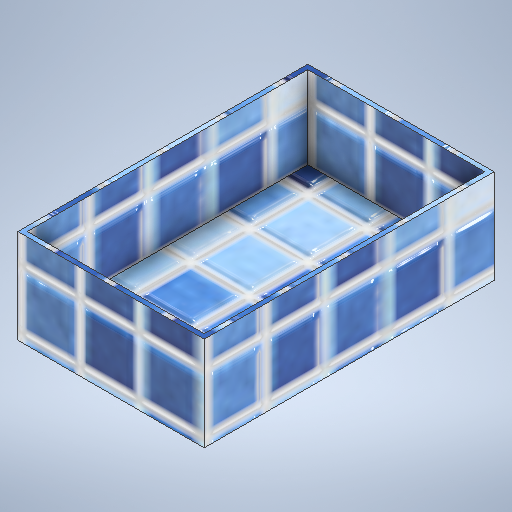
# Autodesk Inventor part: body
Saved by Autodesk Inventor 2025.2 (Build 292293000, 293)
## iProperties
Created: 2025-08-16
Part Number: body
Material: Generic
Document SubType Name: Modeling
Designer: pakiyan
Density: 1 g/cm^3
Appearance: Default
Author: pakiyan
Autodesk Inventor part; units mm, degrees
ref_plane "YZ Plane" through (0, 0, 0) normal (1, 0, 0) x (0, 1, 0)
ref_plane "XZ Plane" through (0, 0, 0) normal (0, 1, 0) x (-1, 0, 0)
ref_plane "XY Plane" through (0, 0, 0) normal (0, 0, 1) x (1, 0, 0)
sketch "Sketch1" plane through (0, 0, 0) normal (0, 1, 0) x (-1, 0, 0)
  line L0 (37.6, 59.6) -> (-37.6, 59.6)
  line L1 (-37.6, 59.6) -> (-37.6, -59.6)
  line L2 (-37.6, -59.6) -> (37.6, -59.6)
  line L3 (37.6, -59.6) -> (37.6, 59.6)
  line L4 (37.6, 59.6) -> (-37.6, -59.6) construction
  line L5 (-37.6, 59.6) -> (37.6, -59.6) construction
  line L6 (39.6, 61.6) -> (-39.6, 61.6)
  line L7 (-39.6, 61.6) -> (-39.6, -61.6)
  line L8 (-39.6, -61.6) -> (39.6, -61.6)
  line L9 (39.6, -61.6) -> (39.6, 61.6)
  point P0 (0, 0)
  dimension "d0" = 119.2
  dimension "d1" = 75.2
  dimension "d2" = 2
  dimension "d3" = 2
  dimension "d4" = 2
  dimension "d5" = 2
  constraints: 20 end point, 4 parallel, 2 horizontal, 2 midpoint, 2 perpendicular
  measures "d0" distance of L0.end L1.end
  measures "d1" distance of L1.end L2.end
  measures "d2" distance between parallel lines of L3 L9
  measures "d3" distance between parallel lines of L8 L2
  measures "d4" distance between parallel lines of L7 L1
  measures "d5" distance between parallel lines of L0 L6
extrude "Extrusion1" add sketch "Sketch1" along normal blind 35
sketch "Sketch4" plane through (0, 0, 0) normal (0, -1, 0) x (1, 0, 0)
  line L0 (-39.6, 61.6) -> (39.6, 61.6) projected
  line L1 (39.6, 61.6) -> (-39.6, 61.6)
  line L2 (-39.6, 61.6) -> (-39.6, -61.6)
  line L3 (-39.6, -61.6) -> (39.6, -61.6)
  line L4 (39.6, -61.6) -> (39.6, 61.6)
  point P0 (0, 0)
  point P1 (-39.6, 61.6)
  constraints: 8 end point, 2 parallel, 1 horizontal, 1 perpendicular
extrude "Extrusion2" add sketch "Sketch4" along normal blind 5
body "Solid1"
